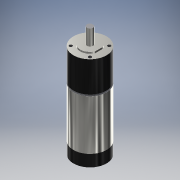
# Autodesk Inventor part: IG-42GM_motor
Saved by Autodesk Inventor 2017 (Build 210142000, 142)
## iProperties
Created: 2015-09-01
Part Number: IG-42GM_motor
Material: 일반
Document SubType Name: Modeling
Designer: EUNSOL
Density: 3.21831 g/cm^3
Appearance: 기본값
Mass: 551 g
Surface Area: 198.39 cm^2
Volume: 171.208 cm^3
Author: EUNSOL
Autodesk Inventor part; units mm, degrees
ref_plane "YZ Plane" through (0, 0, 0) normal (1, 0, 0) x (0, 1, 0)
ref_plane "XZ Plane" through (0, 0, 0) normal (0, 1, 0) x (-1, 0, 0)
ref_plane "XY Plane" through (0, 0, 0) normal (0, 0, 1) x (1, 0, 0)
sketch "스케치1" plane through (0, 0, 0) normal (0, 0, 1) x (1, 0, 0)
  circle A0 centre (0, 0) radius 21.2
  dimension "d0" = 42.4
  constraints: 1 centre point, 1 coincident
  measures "d0" diameter of A0
extrude "돌출1" add sketch "스케치1" along normal blind 39.2
sketch "스케치2" plane through (0, 0, 0) normal (0, 0, -1) x (-1, 0, 0)
  circle A0 centre (0, 0) radius 21
  dimension "d5" = 42
  constraints: 1 centre point, 1 coincident
  measures "d5" diameter of A0
extrude "돌출2" add sketch "스케치2" along normal blind 2
sketch "스케치3" plane through (0, 0, -2) normal (0, 0, -1) x (-1, 0, 0)
  circle A0 centre (0, 0) radius 21.2
  constraints: 1 centre point, 1 coincident
extrude "돌출3" add sketch "스케치3" along normal blind 64
sketch "스케치4" plane through (0, 0, -66) normal (0, 0, -1) x (-1, 0, 0)
  circle A0 centre (0, 0) radius 21.15
  dimension "d19" = 42.3
  constraints: 1 centre point, 1 coincident
  measures "d19" diameter of A0
extrude "돌출4" add sketch "스케치4" along normal blind 15
sketch "스케치5" plane through (0, 0, 39.2) normal (0, 0, 1) x (1, 0, 0)
  circle A0 centre (0, 0) radius 12.5
  line L0 (0, 0) -> (11.5, 0)
  line L1 (11.5, 0) -> (11.5, 4.899)
  line L2 (11.5, 0) -> (11.5, -4.899)
  line L3 (0, 0) -> (-11.5, 0)
  line L4 (-11.5, 0) -> (-11.5, 4.899)
  line L5 (-11.5, 0) -> (-11.5, -4.899)
  dimension "d10" = 25
  dimension "d20" = 11.5
  dimension "d21" = 11.5
  constraints: 12 end point, 4 point on circle, 3 point on line, 2 perpendicular, 1 centre point, 1 coincident, 1 horizontal
  measures "d10" diameter of A0
  measures "d20" distance of L0.start L0.end
  measures "d21" distance of L0.start L3.end
extrude "돌출5" add sketch "스케치5" along normal blind 2 contours L1 L0 L3 L4 A0 | A0 L5 L3 L0 L2
sketch "스케치6" plane through (0, 0, 41.2) normal (0, 0, 1) x (-1, 0, 0)
  circle A0 centre (0, 0) radius 4
  dimension "d13" = 8
  constraints: 1 centre point, 1 coincident
  measures "d13" diameter of A0
extrude "돌출6" add sketch "스케치6" along normal blind 8
sketch "스케치7" plane through (0, 0, 49.2) normal (0, 0, 1) x (1, 0, 0)
  line L0 (0, 0) -> (0, 3.5)
  line L1 (0, 3.5) -> (1.9365, 3.5)
  circle A0 centre (0, 0) radius 4 projected
  line L2 (0, 3.5) -> (-1.9365, 3.5)
  arc A1 (-1.9365, 3.5) -> (1.9365, 3.5) centre (0, 0) ccw
  dimension "d16" = 3.5
  constraints: 6 end point, 4 point on circle, 1 centre point, 1 coincident, 1 perpendicular, 1 point on line, 1 vertical
  measures "d16" distance of L0.start L0.end
extrude "돌출7" add sketch "스케치7" along normal blind 12 contours L1 A0 L2 picked at (-0.0999, -1.4777)
sketch "스케치8" plane through (0, 0, 39.2) normal (0, 0, 1) x (1, 0, 0)
  arc A0 (11.5, 4.899) -> (-11.5, 4.899) centre (0, 0) ccw projected
  line L0 (11.5, 4.899) -> (11.5, -4.899) projected
  arc A1 (-11.5, -4.899) -> (11.5, -4.899) centre (0, 0) ccw projected
  line L1 (-11.5, -4.899) -> (-11.5, 4.899) projected
  circle A2 centre (0, 0) radius 21.2 projected
  line L2 (0, 0) -> (12.3744, 12.3744)
  line L3 (0, 0) -> (17.5, 0) construction
  circle A3 centre (12.3744, 12.3744) radius 2
  circle A4 centre (-12.3744, 12.3744) radius 2
  circle A5 centre (-12.3744, -12.3744) radius 2
  circle A6 centre (12.3744, -12.3744) radius 2
  dimension "d22" = 17.5
  dimension "d23" = 45
  dimension "d24" = 4
  dimension "d27" = 360
  constraints: 4 centre point, 4 end point, 1 coincident, 1 equal length, 1 horizontal, 9 other
  measures "d22" distance of L2.start L2.end
  measures "d23" angle of L3 L2
  measures "d24" diameter of A3
extrude "돌출8" cut sketch "스케치8" against normal blind 6 contours A3 | A4 | A5 | A6
thread "스레드1" size "M4x0.7" class "6H" standard "ANSI Metric M Profile" full length
thread "스레드2" size "M4x0.7" class "6H" standard "ANSI Metric M Profile" full length
thread "스레드3" size "M4x0.7" class "6H" standard "ANSI Metric M Profile" full length
thread "스레드4" size "M4x0.7" class "6H" standard "ANSI Metric M Profile" full length
